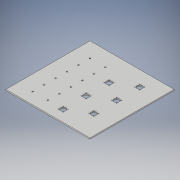
# Autodesk Inventor part: panel
Saved by Autodesk Inventor 2017 (Build 210142000, 142)
## iProperties
Created: 2016-07-20
Part Number: panel
Material: Generic
Document SubType Name: Modeling
Designer: Zuhra Abdurashidova
Density: 1 g/cm^3
Appearance: Default
Author: Zuhra Abdurashidova
Autodesk Inventor part; units mm, degrees
ref_plane "YZ Plane" through (0, 0, 0) normal (1, 0, 0) x (0, 1, 0)
ref_plane "XZ Plane" through (0, 0, 0) normal (0, 1, 0) x (-1, 0, 0)
ref_plane "XY Plane" through (0, 0, 0) normal (0, 0, 1) x (1, 0, 0)
sketch "Sketch1" plane through (0, 0, 0) normal (0, 1, 0) x (-1, 0, 0)
  line L0 (0, 0) -> (-440, 0)
  line L1 (-440, 0) -> (-440, -440)
  line L2 (-440, -440) -> (0, -440)
  line L3 (0, -440) -> (0, 0)
  line L4 (-76.8377, -361.5) -> (-76.8377, -358.5)
  arc A0 (-76.8377, -358.5) -> (-76.8377, -361.5) centre (-80, -360) ccw
  line L5 (-156.8377, -361.5) -> (-156.8377, -358.5)
  arc A1 (-156.8377, -358.5) -> (-156.8377, -361.5) centre (-160, -360) ccw
  line L6 (-76.8377, -301.5) -> (-76.8377, -298.5)
  arc A2 (-76.8377, -298.5) -> (-76.8377, -301.5) centre (-80, -300) ccw
  line L7 (-156.8377, -301.5) -> (-156.8377, -298.5)
  arc A3 (-156.8377, -298.5) -> (-156.8377, -301.5) centre (-160, -300) ccw
  line L8 (-76.8377, -241.5) -> (-76.8377, -238.5)
  arc A4 (-76.8377, -238.5) -> (-76.8377, -241.5) centre (-80, -240) ccw
  line L9 (-156.8377, -241.5) -> (-156.8377, -238.5)
  arc A5 (-156.8377, -238.5) -> (-156.8377, -241.5) centre (-160, -240) ccw
  line L10 (-76.8377, -181.5) -> (-76.8377, -178.5)
  arc A6 (-76.8377, -178.5) -> (-76.8377, -181.5) centre (-80, -180) ccw
  line L11 (-156.8377, -181.5) -> (-156.8377, -178.5)
  arc A7 (-156.8377, -178.5) -> (-156.8377, -181.5) centre (-160, -180) ccw
  line L12 (-76.8377, -121.5) -> (-76.8377, -118.5)
  arc A8 (-76.8377, -118.5) -> (-76.8377, -121.5) centre (-80, -120) ccw
  line L13 (-156.8377, -121.5) -> (-156.8377, -118.5)
  arc A9 (-156.8377, -118.5) -> (-156.8377, -121.5) centre (-160, -120) ccw
  line L14 (-76.8377, -61.5) -> (-76.8377, -58.5)
  arc A10 (-76.8377, -58.5) -> (-76.8377, -61.5) centre (-80, -60) ccw
  line L15 (-156.8377, -61.5) -> (-156.8377, -58.5)
  arc A11 (-156.8377, -58.5) -> (-156.8377, -61.5) centre (-160, -60) ccw
  circle A12 centre (-340, -360) radius 14
  circle A13 centre (-340, -360) radius 17.5 construction
  line L16 (-340, -360) -> (-390.216, -360) construction
  line L17 (-340, -360) -> (-300.4396, -360) construction
  line L18 (-340, -360) -> (-352.3744, -372.3744) construction
  line L19 (-340, -360) -> (-327.6256, -372.3744) construction
  line L20 (-340, -360) -> (-327.6256, -347.6256) construction
  line L21 (-340, -360) -> (-353.5956, -346.4044) construction
  circle A14 centre (-352.3744, -347.6256) radius 2
  circle A15 centre (-327.6256, -347.6256) radius 2
  circle A16 centre (-327.6256, -372.3744) radius 2
  circle A17 centre (-352.3744, -372.3744) radius 2
  circle A18 centre (-327.6256, -252.3744) radius 2
  circle A19 centre (-352.3744, -252.3744) radius 2
  circle A20 centre (-340, -240) radius 14
  circle A21 centre (-327.6256, -227.6256) radius 2
  circle A22 centre (-352.3744, -227.6256) radius 2
  circle A23 centre (-327.6256, -132.3744) radius 2
  circle A24 centre (-352.3744, -132.3744) radius 2
  circle A25 centre (-340, -120) radius 14
  circle A26 centre (-327.6256, -107.6256) radius 2
  circle A27 centre (-352.3744, -107.6256) radius 2
  circle A28 centre (-240, -300) radius 14
  circle A29 centre (-240, -300) radius 17.5 construction
  line L22 (-240, -300) -> (-290.216, -300) construction
  line L23 (-240, -300) -> (-200.4396, -300) construction
  line L24 (-240, -300) -> (-252.3744, -312.3744) construction
  line L25 (-240, -300) -> (-227.6256, -312.3744) construction
  line L26 (-240, -300) -> (-227.6256, -287.6256) construction
  line L27 (-240, -300) -> (-253.5956, -286.4044) construction
  circle A30 centre (-252.3744, -287.6256) radius 2
  circle A31 centre (-227.6256, -287.6256) radius 2
  circle A32 centre (-227.6256, -312.3744) radius 2
  circle A33 centre (-252.3744, -312.3744) radius 2
  line L28 (-240, -180) -> (-290.216, -180) construction
  circle A34 centre (-252.3744, -192.3744) radius 2
  line L29 (-240, -180) -> (-252.3744, -192.3744) construction
  circle A35 centre (-252.3744, -167.6256) radius 2
  line L30 (-240, -180) -> (-253.5956, -166.4044) construction
  line L31 (-240, -180) -> (-227.6256, -192.3744) construction
  circle A36 centre (-227.6256, -192.3744) radius 2
  line L32 (-240, -180) -> (-227.6256, -167.6256) construction
  circle A37 centre (-240, -180) radius 14
  circle A38 centre (-240, -180) radius 17.5 construction
  circle A39 centre (-227.6256, -167.6256) radius 2
  line L33 (-240, -180) -> (-200.4396, -180) construction
  line L34 (-240, -60) -> (-290.216, -60) construction
  circle A40 centre (-252.3744, -72.3744) radius 2
  line L35 (-240, -60) -> (-252.3744, -72.3744) construction
  circle A41 centre (-252.3744, -47.6256) radius 2
  line L36 (-240, -60) -> (-253.5956, -46.4044) construction
  line L37 (-240, -60) -> (-227.6256, -72.3744) construction
  circle A42 centre (-227.6256, -72.3744) radius 2
  line L38 (-240, -60) -> (-227.6256, -47.6256) construction
  circle A43 centre (-240, -60) radius 14
  circle A44 centre (-240, -60) radius 17.5 construction
  circle A45 centre (-227.6256, -47.6256) radius 2
  line L39 (-240, -60) -> (-200.4396, -60) construction
  dimension "d0" = 440
  dimension "d1" = 440
  dimension "d107" = 3.5
  dimension "d109" = 3
  dimension "d111" = 80
  dimension "d135" = 80
  dimension "d138" = 80
  dimension "d141" = 60
  dimension "d163" = 28
  dimension "d164" = 35
  dimension "d166" = 45
  dimension "d167" = 45
  dimension "d169" = 45
  dimension "d170" = 45
  dimension "d171" = 4
  dimension "d172" = 4
  dimension "d173" = 4
  dimension "d174" = 80
  dimension "d176" = 4
  dimension "d179" = 120
  dimension "d184" = 28
  dimension "d185" = 35
  dimension "d186" = 45
  dimension "d187" = 45
  dimension "d188" = 45
  dimension "d189" = 45
  dimension "d190" = 4
  dimension "d191" = 4
  dimension "d192" = 4
  dimension "d193" = 4
  dimension "d194" = 200
  dimension "d195" = 140
  dimension "d198" = 120
  dimension "d205" = 100
  constraints: 80 end point, 46 centre point, 44 point on circle, 12 coincident, 6 horizontal, 4 point on line, 4 vertical, 2 parallel, 1 perpendicular, 123 other
  measures "d0" distance of L1.end L2.end
  measures "d1" distance of L0.end L1.end
  measures "d107" radius of A0
  measures "d109" distance of L4.start L4.end
  measures "d111" distance from line of L2 A0.centre
  measures "d135" distance from line of A0.centre L3
  measures "d138" distance of L4.start L5.start
  measures "d141" distance of L4.start L6.start
  measures "d163" diameter of A12
  measures "d164" diameter of A13
  measures "d166" angle of L18 L16
  measures "d167" angle of L19 L17
  measures "d169" angle of L20 L17
  measures "d170" angle of L21 L16
  measures "d171" diameter of A14
  measures "d172" diameter of A15
  measures "d173" diameter of A16
  measures "d174" distance from line of L2 A12.centre
  measures "d176" diameter of A17
  measures "d179" distance of A16.centre A18.centre
  measures "d184" diameter of A28
  measures "d185" diameter of A29
  measures "d186" angle of L24 L22
  measures "d187" angle of L25 L23
  measures "d188" angle of L26 L23
  measures "d189" angle of L27 L22
  measures "d190" diameter of A30
  measures "d191" diameter of A31
  measures "d192" diameter of A32
  measures "d193" diameter of A33
  measures "d194" distance from line of L1 A28.centre
  measures "d195" distance from line of L2 A28.centre
  measures "d198" distance of L22.start L28.start
  measures "d205" distance from line of L1 L16.start
extrude "Extrusion5" add sketch "Sketch1" along normal blind 6
body "Solid5"
